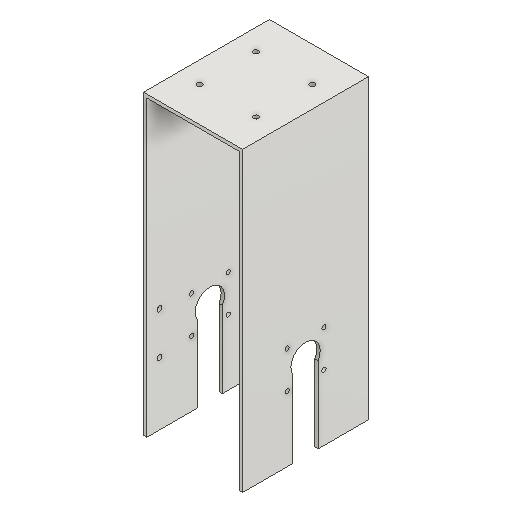
# Autodesk Inventor part: CShape
Saved by Autodesk Inventor 2022 (Build 260153000, 153)
## iProperties
Created: 2024-07-02
Part Number: CShape
Material: Generic
Document SubType Name: Modeling
Designer: LaptopJR
Density: 1 g/cm^3
Appearance: Steel
Author: LaptopJR
Autodesk Inventor part; units mm, degrees
ref_plane "YZ Plane" through (0, 0, 0) normal (1, 0, 0) x (0, 1, 0)
ref_plane "XZ Plane" through (0, 0, 0) normal (0, 1, 0) x (-1, 0, 0)
sketch "Sketch1" plane through (0, 0, 0) normal (0, 0, 1) x (1, 0, 0)
  line L0 (0, 0) -> (0, 350)
  line L1 (0, 350) -> (110, 350)
  line L2 (110, 350) -> (110, 0)
  line L3 (114, 0) -> (114, 354)
  line L4 (114, 354) -> (-4, 354)
  line L5 (-4, 354) -> (-4, 0)
  line L6 (-4, 0) -> (0, 0)
  line L7 (110, 0) -> (114, 0)
  dimension "d0" = 350
  dimension "d1" = 110
  dimension "d2" = 4
  constraints: 16 end point, 3 perpendicular, 2 horizontal, 1 parallel, 1 vertical, 2 other
  measures "d0" distance of L0.start L0.end
  measures "d1" distance of L0.end L1.end
  measures "d2" distance between parallel lines of L1 L4
extrude "Extrusion1" add sketch "Sketch1" along normal blind 150
sketch "Sketch2" plane through (-4, 0, 0) normal (-1, 0, 0) x (0, 0, 1)
  line L0 (0, 354) -> (150, 354) projected
  line L1 (0, 0) -> (150, 0) projected
  line L2 (75, 0) -> (75, 100) construction
  circle A0 centre (75, 100) radius 17.5
  line L3 (60, 0) -> (60, 90.9861)
  line L4 (90, 0) -> (90, 90.9861)
  circle A1 centre (100, 100) radius 31 construction
  line L5 (75, 100) -> (53.0797, 121.9203) construction
  circle A2 centre (53.0797, 121.9203) radius 2.55
  circle A3 centre (53.0797, 78.0797) radius 2.55
  circle A4 centre (96.9203, 78.0797) radius 2.55
  circle A5 centre (96.9203, 121.9203) radius 2.55
  point P0 (60, 0)
  point P1 (90, 0)
  dimension "d5" = 100
  dimension "d6" = 15
  dimension "d7" = 15
  dimension "d12" = 35
  dimension "d13" = 62
  dimension "d23" = 5.1
  dimension "d26" = 360
  constraints: 8 end point, 6 centre point, 3 coincident, 2 parallel, 2 point on circle, 1 midpoint, 1 vertical, 9 other
  measures "d5" distance of L2.start L2.end
  measures "d6" distance between parallel lines of L2 L3
  measures "d7" distance between parallel lines of L2 L4
  measures "d12" diameter of A0
  measures "d13" diameter of A1
  measures "d23" diameter of A2
extrude "Extrusion2" cut sketch "Sketch2" against normal blind 200
sketch "Sketch4" plane through (-4, 0, 0) normal (-1, 0, 0) x (0, 0, 1)
  arc A0 (90, 90.9861) -> (60, 90.9861) centre (75, 100) ccw construction
  line L0 (15, 75) -> (135, 75) construction
  line L1 (135, 75) -> (135, 125) construction
  line L2 (135, 125) -> (15, 125) construction
  line L3 (15, 125) -> (15, 75) construction
  line L4 (15, 75) -> (135, 125) construction
  line L5 (135, 75) -> (15, 125) construction
  circle A1 centre (15, 125) radius 3.05
  circle A2 centre (15, 75) radius 3.05
  circle A3 centre (135, 75) radius 3.05
  circle A4 centre (135, 125) radius 3.05
  point P0 (0, 0)
  dimension "d33" = 120
  dimension "d34" = 50
  dimension "d35" = 6.1
  constraints: 12 end point, 4 centre point, 4 coincident, 3 equal radius, 2 midpoint, 2 parallel, 1 horizontal, 1 perpendicular
  measures "d33" distance of L2.end L1.end
  measures "d34" distance of L1.end L0.end
  measures "d35" diameter of A1
extrude "Extrusion4" cut sketch "Sketch4" against normal blind 5
ref_plane "Work Plane1" through (55, 0, 0) normal (1, 0, 0) x (0, 0, -1)
sketch "Sketch5" plane through (-4, 354, 0) normal (0, 1, 0) x (1, 0, 0)
  line L0 (118, 0) -> (0, 0) projected
  line L1 (0, 0) -> (0, -150) projected
  line L2 (118, -150) -> (0, -150) projected
  line L3 (118, 0) -> (118, -150) projected
  line L4 (4, -150) -> (114, -150) projected
  line L5 (59, -150) -> (59, 0) construction
  line L6 (4, 0) -> (114, 0) projected
  circle A0 centre (59, -75) radius 5
  circle A1 centre (59, -75) radius 47.5 construction
  line L7 (59, -75) -> (11.5, -75) construction
  line L8 (59, -75) -> (25.4124, -108.5876) construction
  circle A2 centre (25.4124, -108.5876) radius 3.05
  circle A3 centre (92.5876, -108.5876) radius 3.05
  circle A4 centre (92.5876, -41.4124) radius 3.05
  circle A5 centre (25.4124, -41.4124) radius 3.05
  dimension "d38" = 10
  dimension "d41" = 95
  dimension "d42" = 6.1
  dimension "d43" = 45
  dimension "d46" = 360
  constraints: 6 centre point, 6 end point, 3 midpoint, 2 coincident, 2 point on circle, 1 horizontal, 9 other
  measures "d38" diameter of A0
  measures "d41" diameter of A1
  measures "d42" diameter of A2
  measures "d43" angle of L7 L8
extrude "Extrusion5" cut sketch "Sketch5" against normal blind 20 contours A2 | A3 | A4 | A5
body "Solid1"
